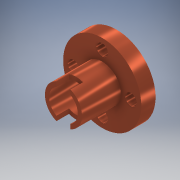
# Autodesk Inventor part: nakretka tr08
Saved by Autodesk Inventor 2017 SP1 (Build 210196100, 196)
## iProperties
Created: 2017-03-01
Part Number: nakretka tr08
Material: Ogólny
Document SubType Name: Modeling
Designer: user
Density: 1 g/cm^3
Appearance: Gorący metal 1400F
Author: user
Autodesk Inventor part; units mm, degrees
ref_plane "YZ Plane" through (0, 0, 0) normal (1, 0, 0) x (0, 1, 0)
ref_plane "XZ Plane" through (0, 0, 0) normal (0, 1, 0) x (-1, 0, 0)
ref_plane "XY Plane" through (0, 0, 0) normal (0, 0, 1) x (1, 0, 0)
sketch "Szkic1" plane through (0, 0, 0) normal (0, 1, 0) x (-1, 0, 0)
  circle A0 centre (0, 0) radius 10.875
  circle A1 centre (0, 0) radius 4
  point P0 (8, 0)
  point P1 (0, -8)
  point P2 (-8, 0)
  point P3 (0, 8)
  dimension "d0" = 21.75
  dimension "d1" = 8
  dimension "d2" = 8
  dimension "d5" = 360
  constraints: 2 centre point, 2 coincident, 5 other
  measures "d0" diameter of A0
  measures "d1" diameter of A1
  measures "d2" distance of point (0, 0) point (8, 0)
extrude "Wyciągnięcie proste1" add sketch "Szkic1" along normal blind 4
sketch "Szkic2" plane through (0, 4, 0) normal (0, 1, 0) x (1, 0, 0)
  circle A0 centre (0, 0) radius 4 projected
  circle A1 centre (0, 0) radius 10.875 projected
  point P0 (-8, 0)
  point P1 (0, -8)
  point P2 (8, 0)
  point P3 (0, 8)
  dimension "d11" = 360
  dimension "d20" = 8
  constraints: 1 horizontal alignment, 5 other
  measures "d20" distance of point (-8, 0) point (0, 0)
hole "Otwór1" at (-8, 4, 0) at (0, 4, 8) at (8, 4, 0) at (0, 4, -8) direction (0, -1, 0) diameter 3.2 end through all
sketch "Szkic3" plane through (0, 0, 0) normal (0, -1, 0) x (1, 0, 0)
  circle A0 centre (0, 0) radius 5.17
  circle A1 centre (0, 0) radius 4 projected
  dimension "d21" = 10.34
  constraints: 1 centre point
  measures "d21" diameter of A0
extrude "Wyciągnięcie proste2" add sketch "Szkic3" along normal blind 10.8
sketch "Szkic4" plane through (0, 0, 0) normal (1, 0, 0) x (0, 1, 0)
  line L0 (-10.8, 5.17) -> (-7.3, 5.17)
  line L1 (-7.3, 5.17) -> (-7.3, -5.17)
  line L2 (-7.3, -5.17) -> (-10.8, -5.17)
  line L3 (-10.8, -5.17) -> (-10.8, 5.17)
  line L4 (0, -5.17) -> (0, 5.17) projected
  line L5 (-10.8, -4) -> (-10.8, 4) projected
  line L6 (0, 5.17) -> (-10.8, 5.17) projected
  line L7 (0, -5.17) -> (-10.8, -5.17) projected
  line L8 (-10.8, 0) -> (4, 0)
  line L9 (4, -10.875) -> (4, 10.875) projected
  point P0 (0, 0)
  dimension "d24" = 10.34
  dimension "d25" = 7.3
  dimension "d26" = 10.34
  constraints: 10 end point, 3 midpoint, 2 parallel, 1 coincident, 1 horizontal, 1 perpendicular, 1 other
  measures "d24" distance of L0.end L1.end
  measures "d25" distance between parallel lines of L1 L4
  measures "d26" distance between parallel lines of L7 L6
extrude "Wyciągnięcie proste3" cut sketch "Szkic4" along normal mid plane 3.9 contours L0 L1 L8 L3 | L1 L2 L3 L8
equation "\"d24\" = d26"
